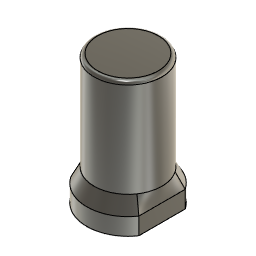
secondary_007mm_abxy_4x v2 (Autodesk Fusion 360 design; units mm, degrees)
Autodesk Fusion 360 part; units mm, degrees
other "Base Mesh Feature1"
sketch "Sketch1" plane through (0, 0, 0) normal (0, 0, 1) x (1, 0, 0)
  circle A0 centre (0, 0) radius 1
  dimension "d1" = 2
  constraint coincident A0.centre origin
  measures "d1" diameter of A0
other "Modify1"
sketch "Sketch2" plane through (0, 0, 0) normal (0, 0, 1) x (1, 0, 0)
  circle A0 centre (0, 0) radius 5.8091
  line L0 (4.8004, -3.4792) -> (6.0576, -3.4792)
  line L1 (6.0576, -3.4792) -> (6.0576, 3.507)
  line L2 (6.0576, 3.507) -> (4.8004, 3.507)
  line L3 (4.8004, 3.507) -> (4.8004, -3.4792)
  line L4 (0, -8) -> (0, 8) construction
  line L5 (0, -8) -> (0, 8) construction
  line L6 (-4.8004, 3.507) -> (-4.8004, -3.4792)
  line L7 (-4.8004, -3.4792) -> (-6.0576, -3.4792)
  line L8 (-6.0576, -3.4792) -> (-6.0576, 3.507)
  line L9 (-6.0576, 3.507) -> (-4.8004, 3.507)
  constraint coincident A0.centre origin
  constraint horizontal L0
  constraint vertical L1
  constraint horizontal L2
  constraint vertical L3
  constraint vertical L4
  constraint symmetric L0.start L4 L6.end
  constraint symmetric L0.end L4 L7.end
  constraint symmetric L1.end L4 L8.end
  constraint symmetric L2.end L4 L6.start
  constraint symmetric L5.start L4 L4.start
  constraint symmetric L5.end L4 L4.end
extrude "Extrude1" add sketch "Sketch1" sketch "Sketch2" along normal blind 2.4 of sketch 2 contours A0 L3 L6 makes body 1
ref_plane "WorkPlane1" through (0, 0, 18.25) normal (0, 0, 1) x (1, 0, 0)
sketch "Sketch3" plane through (0, 0, 18.25) normal (0, 0, 1) x (1, 0, 0)
  circle A0 centre (0, 0) radius 4.7834
  constraint coincident A0.centre origin
extrude "Extrude2" add sketch "Sketch3" against normal blind 13.85 separate body makes body 2
loft "Loft1" add section 1 face at (1.4197, 1.3168, 2.4) section 2 face at (-1.3835, -0.0158, 4.4) on bodies 1 2 bodies 1 2
fillet "Fillet1" radius 0.5 1 edges at (-4.4597, -1.7297, 18.25) on bodies 1
named bodies: "secondary_007mm_abxy_4x (1)"
